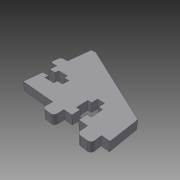
# Autodesk Inventor part: z_axis_top_brace
Saved by Autodesk Inventor 2014 (Build 180170000, 170)
## iProperties
Created: 2013-12-08
Part Number: z_axis_top_brace
Material: Generic
Document SubType Name: Modeling
Designer: buben
Density: 1 g/cm^3
Appearance: Default
Author: buben
Autodesk Inventor part; units mm, degrees
ref_plane "YZ Plane" through (0, 0, 0) normal (1, 0, 0) x (0, 1, 0)
ref_plane "XZ Plane" through (0, 0, 0) normal (0, 1, 0) x (-1, 0, 0)
ref_plane "XY Plane" through (0, 0, 0) normal (0, 0, 1) x (1, 0, 0)
sketch "Sketch1" plane through (0, 0, 0) normal (0, 0, 1) x (1, 0, 0)
  line L0 (0, 50) -> (0, 0)
  line L1 (0, 0) -> (60, 0)
  line L2 (60, 0) -> (60, 18)
  line L3 (60, 18) -> (4, 50)
  line L4 (4, 50) -> (0, 50)
  dimension "d0" = 60
  dimension "d1" = 50
  dimension "d2" = 4
  dimension "d3" = 18
  constraints: 10 end point, 2 parallel, 1 perpendicular, 1 vertical
  measures "d0" distance of L0.end L1.end
  measures "d1" distance of L0.start L0.end
  measures "d2" distance of L3.end L0.start
  measures "d3" distance of L1.end L2.end
extrude "Extrusion1" add sketch "Sketch1" along normal blind 6
sketch "Sketch2" plane through (0, 0, 6) normal (0, 0, 1) x (1, 0, 0)
  line L0 (0, 50) -> (0, 0) projected
  line L1 (0, 0) -> (60, 0) projected
  line L2 (37.75, 16.3) -> (42.25, 16.3)
  line L3 (42.25, 0) -> (37.75, 0)
  line L4 (44.75, 12.3) -> (44.75, 5)
  line L5 (35.25, 5) -> (35.25, 12.3)
  line L6 (16.3, 17.25) -> (16.3, 12.75)
  line L7 (0, 12.75) -> (0, 17.25)
  line L8 (5, 19.75) -> (12.3, 19.75)
  line L9 (12.3, 10.25) -> (5, 10.25)
  line L10 (0, 17.25) -> (5, 17.25)
  line L11 (12.3, 17.25) -> (16.3, 17.25)
  line L12 (16.3, 12.75) -> (12.3, 12.75)
  line L13 (5, 12.75) -> (0, 12.75)
  line L14 (5, 10.25) -> (5, 12.75)
  line L15 (5, 17.25) -> (5, 19.75)
  line L16 (12.3, 19.75) -> (12.3, 17.25)
  line L17 (12.3, 12.75) -> (12.3, 10.25)
  line L18 (35.25, 12.3) -> (37.75, 12.3)
  line L19 (42.25, 12.3) -> (44.75, 12.3)
  line L20 (44.75, 5) -> (42.25, 5)
  line L21 (37.75, 5) -> (35.25, 5)
  line L22 (37.75, 0) -> (37.75, 5)
  line L23 (37.75, 12.3) -> (37.75, 16.3)
  line L24 (42.25, 16.3) -> (42.25, 12.3)
  line L25 (42.25, 5) -> (42.25, 0)
  point P0 (16.3, 15)
  point P1 (0, 25)
  point P2 (40, 16.3)
  dimension "d6" = 4.5
  dimension "d7" = 4.5
  dimension "d8" = 2.5
  dimension "d9" = 2.5
  dimension "d10" = 2.5
  dimension "d11" = 2.5
  dimension "d12" = 5
  dimension "d13" = 4
  dimension "d14" = 7.3
  dimension "d15" = 5
  dimension "d16" = 4
  dimension "d17" = 7.3
  dimension "d34" = 15
  dimension "d35" = 40
  constraints: 48 end point, 20 parallel, 10 collinear, 8 perpendicular, 6 horizontal, 3 midpoint
  measures "d6" distance of L2.start L2.end
  measures "d7" distance of L6.start L6.end
  measures "d8" distance of L5.end L18.end
  measures "d9" distance of L19.start L4.start
  measures "d10" distance of L12.end L9.start
  measures "d11" distance of L8.end L11.start
  measures "d12" distance of L13.start L7.start
  measures "d13" distance of L6.end L12.end
  measures "d14" distance of L9.start L9.end
  measures "d15" distance of L3.end L21.start
  measures "d16" distance of L18.end L2.start
  measures "d17" distance of L5.start L5.end
  measures "d34" distance from line of L1 point (16.3, 15)
  measures "d35" distance from line of L0 point (40, 16.3)
extrude "Extrusion2" cut sketch "Sketch2" against normal blind 6
sketch "Sketch4" plane through (0, 0, 6) normal (0, 0, 1) x (1, 0, 0)
  line L0 (42.25, 0) -> (60, 0) projected
  line L1 (0, 50) -> (0, 17.25) projected
  line L2 (16.3, 17.25) -> (16.3, 12.75) projected
  line L3 (0, 0) -> (37.75, 0) projected
  line L4 (37.75, 16.3) -> (42.25, 16.3) projected
  line L5 (0, 30.5) -> (-4, 30.5)
  line L6 (-6, 28.5) -> (-6, 24.5)
  line L7 (-4, 22.5) -> (0, 22.5)
  line L8 (0, 22.5) -> (0, 30.5)
  line L9 (24.5, 0) -> (32.5, 0)
  line L10 (32.5, 0) -> (32.5, -4)
  line L11 (30.5, -6) -> (26.5, -6)
  line L12 (24.5, -4) -> (24.5, 0)
  line L13 (47.5, 0) -> (55.5, 0)
  line L14 (55.5, 0) -> (55.5, -4)
  line L15 (53.5, -6) -> (49.5, -6)
  line L16 (47.5, -4) -> (47.5, 0)
  arc A0 (-4, 30.5) -> (-6, 28.5) centre (-4, 28.5) ccw
  arc A1 (-6, 24.5) -> (-4, 22.5) centre (-4, 24.5) ccw
  arc A2 (24.5, -4) -> (26.5, -6) centre (26.5, -4) ccw
  arc A3 (30.5, -6) -> (32.5, -4) centre (30.5, -4) ccw
  arc A4 (47.5, -4) -> (49.5, -6) centre (49.5, -4) ccw
  arc A5 (53.5, -6) -> (55.5, -4) centre (53.5, -4) ccw
  point P0 (16.3, 15)
  point P1 (40, 16.3)
  dimension "d36" = 2
  dimension "d37" = 8
  dimension "d38" = 6
  dimension "d39" = 8
  dimension "d40" = 8
  dimension "d41" = 6
  dimension "d42" = 15
  dimension "d43" = 7.5
  dimension "d44" = 7.5
  constraints: 24 end point, 12 point on circle, 12 tangent, 6 centre point, 6 parallel, 5 equal radius, 3 horizontal, 3 perpendicular, 3 point on line, 2 midpoint, 1 collinear
  measures "d36" radius of A0
  measures "d37" distance between parallel lines of L5 L7
  measures "d38" distance between parallel lines of L1 L6
  measures "d39" distance between parallel lines of L10 L12
  measures "d40" distance between parallel lines of L14 L16
  measures "d41" distance between parallel lines of L0 L15
  measures "d42" distance between parallel lines of L10 L16
  measures "d43" distance from line of point (16.3, 15) L7
  measures "d44" distance from line of point (40, 16.3) L10
extrude "Extrusion4" add sketch "Sketch4" against normal blind 6
body "Solid1"
